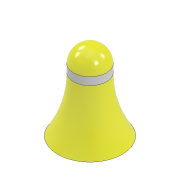
# Autodesk Inventor part: cock1
Saved by Autodesk Inventor 2021 (Build 250183000, 183)
## iProperties
Created: 2021-07-24
Part Number: cock1
Material: Generic
Document SubType Name: Modeling
Designer: user
Density: 1 g/cm^3
Appearance: Default
Author: user
Autodesk Inventor part; units mm, degrees
ref_plane "YZ Plane" through (0, 0, 0) normal (1, 0, 0) x (0, 1, 0)
ref_plane "XZ Plane" through (0, 0, 0) normal (0, 1, 0) x (-1, 0, 0)
ref_plane "XY Plane" through (0, 0, 0) normal (0, 0, 1) x (1, 0, 0)
sketch "Sketch1" plane through (0, 0, 0) normal (0, 1, 0) x (-1, 0, 0)
  arc A0 (-19.05, 0) -> (19.05, 0) centre (0, 0) ccw
  line L0 (19.05, 0) -> (-19.05, 0)
  constraints: 2 end point, 2 point on circle, 1 centre point, 1 coincident, 1 horizontal
revolve "Revolution1" add sketch "Sketch1" angle 180 about axis through (-19.05, 0, 0) along (1, 0, 0)
sketch "Sketch2" plane through (0, 0, 0) normal (0, -1, 0) x (1, 0, 0)
  circle A0 centre (0, 0) radius 19.05
  constraints: 1 centre point, 1 coincident
extrude "Extrusion1" add sketch "Sketch2" along normal blind 8.89
sketch "Sketch3" plane through (0, 0, 0) normal (1, 0, 0) x (0, 1, 0)
  line L0 (-8.89, 19.05) -> (-8.89, -19.05) projected
  line L1 (-8.89, 0) -> (-72.39, 0)
  arc A0 (-72.39, 37.2434) -> (-8.89, 19.05) centre (-8.89, 138.9628) ccw
  arc A1 (-72.39, 34.643) -> (-8.89, 16.8363) centre (-8.89, 138.9628) ccw
  line L2 (-8.89, 16.8363) -> (0, 16.8363)
  line L3 (-72.39, 37.2434) -> (-72.39, 34.643)
  line L4 (-8.89, 16.8363) -> (-8.89, 19.05)
  point P0 (0, 0)
  point P1 (-8.89, 16.8363)
  dimension "d4" = 63.5
  constraints: 8 end point, 4 point on circle, 2 centre point, 2 vertical, 1 horizontal, 1 midpoint
  measures "d4" distance of L1.start L1.end
revolve "Revolution2" add sketch "Sketch3" angle 360 about axis through (0, -8.89, 0) along (0, -1, 0)
body "Solid1"
